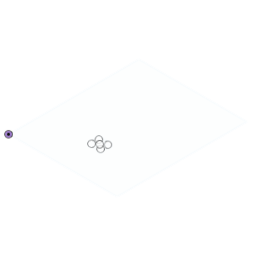
designing_cuts_acrylic_plates (Autodesk Fusion 360 design; units mm, degrees)
part number: 2026-05-25-10-10-53-826
Autodesk Fusion 360 part; units mm, degrees
sketch "Sketch3" plane through (0, 0, 0) normal (0, 0, 1) x (1, 0, 0)
  line L0 (0, 0) -> (225, 0)
  line L1 (225, 0) -> (225, 405)
  line L2 (225, 405) -> (0, 405)
  line L3 (0, 405) -> (0, 0)
  dimension "d6" = 225
  dimension "d7" = 405
  constraint horizontal L0
  constraint vertical L1
  constraint horizontal L2
  constraint vertical L3
  constraint coincident L0.start L3.end
  measures "d6" distance of L1 L3
  measures "d7" distance of L0 L2
sketch "Sketch4" plane through (0, 0, 0) normal (0, 0, 1) x (1, 0, 0)
  line L0 (0, 0) -> (75, 0)
  line L1 (75, 0) -> (75, 81)
  line L2 (75, 81) -> (0, 81)
  line L3 (0, 81) -> (0, 0)
  dimension "d8" = 75
  dimension "d9" = 81
  constraint horizontal L0
  constraint vertical L1
  constraint horizontal L2
  constraint vertical L3
  constraint coincident L0.start L3.end
  measures "d8" distance of L1 L3
  measures "d9" distance of L0 L2
extrude "Extrude1" add sketch "Sketch3" along normal blind 3 makes body 1
sketch "Sketch5" plane through (0, 0, 0) normal (0, 0, 1) x (1, 0, 0)
  line L0 (0, 0) -> (225, 0) construction
  line L1 (225, 0) -> (225, 405) construction
  line L2 (225, 405) -> (0, 405) construction
  line L3 (0, 405) -> (0, 0) construction
  line L4 (0, 81) -> (225, 81) construction
  line L5 (0, 162) -> (225, 162) construction
  line L6 (0, 243) -> (225, 243) construction
  line L7 (0, 324) -> (225, 324) construction
  line L8 (150, 405) -> (150, 0) construction
  line L9 (75, 405) -> (75, 0) construction
  line L10 (22.5, 388.5) -> (52.5, 388.5) construction
  line L11 (52.5, 388.5) -> (52.5, 340.5) construction
  line L12 (52.5, 340.5) -> (22.5, 340.5) construction
  line L13 (22.5, 340.5) -> (22.5, 388.5) construction
  line L14 (127.5, 388.5) -> (127.5, 340.5) construction
  line L15 (97.5, 388.5) -> (127.5, 388.5) construction
  line L16 (97.5, 340.5) -> (97.5, 388.5) construction
  line L17 (127.5, 340.5) -> (97.5, 340.5) construction
  line L18 (202.5, 388.5) -> (202.5, 340.5) construction
  line L19 (172.5, 388.5) -> (202.5, 388.5) construction
  line L20 (172.5, 340.5) -> (172.5, 388.5) construction
  line L21 (202.5, 340.5) -> (172.5, 340.5) construction
  line L22 (22.5, 226.5) -> (52.5, 226.5) construction
  line L23 (22.5, 178.5) -> (22.5, 226.5) construction
  line L24 (52.5, 226.5) -> (52.5, 178.5) construction
  line L25 (52.5, 178.5) -> (22.5, 178.5) construction
  line L26 (97.5, 226.5) -> (127.5, 226.5) construction
  line L27 (97.5, 178.5) -> (97.5, 226.5) construction
  line L28 (127.5, 226.5) -> (127.5, 178.5) construction
  line L29 (127.5, 178.5) -> (97.5, 178.5) construction
  line L30 (172.5, 226.5) -> (202.5, 226.5) construction
  line L31 (172.5, 178.5) -> (172.5, 226.5) construction
  line L32 (202.5, 226.5) -> (202.5, 178.5) construction
  line L33 (202.5, 178.5) -> (172.5, 178.5) construction
  line L34 (22.5, 64.5) -> (52.5, 64.5) construction
  line L35 (22.5, 16.5) -> (22.5, 64.5) construction
  line L36 (52.5, 64.5) -> (52.5, 16.5) construction
  line L37 (52.5, 16.5) -> (22.5, 16.5) construction
  line L38 (97.5, 64.5) -> (127.5, 64.5) construction
  line L39 (97.5, 16.5) -> (97.5, 64.5) construction
  line L40 (127.5, 64.5) -> (127.5, 16.5) construction
  line L41 (127.5, 16.5) -> (97.5, 16.5) construction
  line L42 (172.5, 64.5) -> (202.5, 64.5) construction
  line L43 (172.5, 16.5) -> (172.5, 64.5) construction
  line L44 (202.5, 64.5) -> (202.5, 16.5) construction
  line L45 (202.5, 16.5) -> (172.5, 16.5) construction
  line L46 (52.5, 307.5) -> (52.5, 259.5) construction
  line L47 (22.5, 307.5) -> (52.5, 307.5) construction
  line L48 (22.5, 259.5) -> (22.5, 307.5) construction
  line L49 (52.5, 259.5) -> (22.5, 259.5) construction
  line L50 (97.5, 307.5) -> (127.5, 307.5) construction
  line L51 (127.5, 307.5) -> (127.5, 259.5) construction
  line L52 (97.5, 259.5) -> (97.5, 307.5) construction
  line L53 (127.5, 259.5) -> (97.5, 259.5) construction
  line L54 (172.5, 307.5) -> (202.5, 307.5) construction
  line L55 (172.5, 259.5) -> (172.5, 307.5) construction
  line L56 (202.5, 307.5) -> (202.5, 259.5) construction
  line L57 (202.5, 259.5) -> (172.5, 259.5) construction
  line L58 (22.5, 145.5) -> (52.5, 145.5) construction
  line L59 (22.5, 97.5) -> (22.5, 145.5) construction
  line L60 (52.5, 145.5) -> (52.5, 97.5) construction
  line L61 (52.5, 97.5) -> (22.5, 97.5) construction
  line L62 (97.5, 145.5) -> (127.5, 145.5) construction
  line L63 (97.5, 97.5) -> (97.5, 145.5) construction
  line L64 (127.5, 145.5) -> (127.5, 97.5) construction
  line L65 (127.5, 97.5) -> (97.5, 97.5) construction
  line L66 (172.5, 97.5) -> (172.5, 145.5) construction
  line L67 (172.5, 145.5) -> (202.5, 145.5) construction
  line L68 (202.5, 145.5) -> (202.5, 97.5) construction
  line L69 (202.5, 97.5) -> (172.5, 97.5) construction
  line L70 (22.5, 348.5) -> (52.5, 348.5) construction
  line L71 (25, 340.5) -> (50, 340.5) construction
  line L72 (50, 340.5) -> (50, 372) construction
  line L73 (50, 372) -> (25, 372) construction
  line L74 (25, 372) -> (25, 340.5) construction
  line L75 (26, 358.5) -> (47, 358.5) construction
  line L76 (47, 358.5) -> (47, 341.5) construction
  line L77 (47, 341.5) -> (26, 341.5) construction
  line L78 (26, 341.5) -> (26, 358.5) construction
  line L79 (125, 372) -> (100, 372) construction
  line L80 (100, 372) -> (100, 340.5) construction
  line L81 (125, 340.5) -> (125, 372) construction
  line L82 (122, 358.5) -> (122, 341.5) construction
  line L83 (101, 358.5) -> (122, 358.5) construction
  line L84 (101, 341.5) -> (101, 358.5) construction
  line L85 (122, 341.5) -> (101, 341.5) construction
  line L86 (97.5, 348.5) -> (127.5, 348.5) construction
  line L87 (200, 372) -> (175, 372) construction
  line L88 (175, 372) -> (175, 340.5) construction
  line L89 (200, 340.5) -> (200, 372) construction
  line L90 (197, 358.5) -> (197, 341.5) construction
  line L91 (176, 358.5) -> (197, 358.5) construction
  line L92 (176, 341.5) -> (176, 358.5) construction
  line L93 (197, 341.5) -> (176, 341.5) construction
  line L94 (172.5, 348.5) -> (202.5, 348.5) construction
  line L95 (200, 291) -> (175, 291) construction
  line L96 (176, 277.5) -> (197, 277.5) construction
  line L97 (175, 291) -> (175, 259.5) construction
  line L98 (200, 259.5) -> (200, 291) construction
  line L99 (197, 277.5) -> (197, 260.5) construction
  line L100 (176, 260.5) -> (176, 277.5) construction
  line L101 (197, 260.5) -> (176, 260.5) construction
  line L102 (172.5, 267.5) -> (202.5, 267.5) construction
  line L103 (101, 277.5) -> (122, 277.5) construction
  line L104 (122, 277.5) -> (122, 260.5) construction
  line L105 (122, 260.5) -> (101, 260.5) construction
  line L106 (101, 260.5) -> (101, 277.5) construction
  line L107 (125, 291) -> (100, 291) construction
  line L108 (125, 259.5) -> (125, 291) construction
  line L109 (100, 291) -> (100, 259.5) construction
  line L110 (97.5, 267.5) -> (127.5, 267.5) construction
  line L111 (50, 291) -> (25, 291) construction
  line L112 (25, 291) -> (25, 259.5) construction
  line L113 (50, 259.5) -> (50, 291) construction
  line L114 (26, 277.5) -> (47, 277.5) construction
  line L115 (26, 260.5) -> (26, 277.5) construction
  line L116 (47, 277.5) -> (47, 260.5) construction
  line L117 (22.5, 267.5) -> (52.5, 267.5) construction
  line L118 (47, 260.5) -> (26, 260.5) construction
  line L119 (200, 210) -> (175, 210) construction
  line L120 (176, 196.5) -> (197, 196.5) construction
  line L121 (175, 210) -> (175, 178.5) construction
  line L122 (200, 178.5) -> (200, 210) construction
  line L123 (197, 196.5) -> (197, 179.5) construction
  line L124 (176, 179.5) -> (176, 196.5) construction
  line L125 (197, 179.5) -> (176, 179.5) construction
  line L126 (172.5, 186.5) -> (202.5, 186.5) construction
  line L127 (101, 196.5) -> (122, 196.5) construction
  line L128 (122, 196.5) -> (122, 179.5) construction
  line L129 (122, 179.5) -> (101, 179.5) construction
  line L130 (101, 179.5) -> (101, 196.5) construction
  line L131 (125, 210) -> (100, 210) construction
  line L132 (125, 178.5) -> (125, 210) construction
  line L133 (100, 210) -> (100, 178.5) construction
  line L134 (97.5, 186.5) -> (127.5, 186.5) construction
  line L135 (50, 210) -> (25, 210) construction
  line L136 (25, 210) -> (25, 178.5) construction
  line L137 (50, 178.5) -> (50, 210) construction
  line L138 (26, 196.5) -> (47, 196.5) construction
  line L139 (26, 179.5) -> (26, 196.5) construction
  line L140 (47, 196.5) -> (47, 179.5) construction
  line L141 (22.5, 186.5) -> (52.5, 186.5) construction
  line L142 (47, 179.5) -> (26, 179.5) construction
  line L143 (200, 129) -> (175, 129) construction
  line L144 (176, 115.5) -> (197, 115.5) construction
  line L145 (175, 129) -> (175, 97.5) construction
  line L146 (200, 97.5) -> (200, 129) construction
  line L147 (197, 115.5) -> (197, 98.5) construction
  line L148 (176, 98.5) -> (176, 115.5) construction
  line L149 (197, 98.5) -> (176, 98.5) construction
  line L150 (172.5, 105.5) -> (202.5, 105.5) construction
  line L151 (101, 115.5) -> (122, 115.5) construction
  line L152 (122, 115.5) -> (122, 98.5) construction
  line L153 (122, 98.5) -> (101, 98.5) construction
  line L154 (101, 98.5) -> (101, 115.5) construction
  line L155 (125, 129) -> (100, 129) construction
  line L156 (125, 97.5) -> (125, 129) construction
  line L157 (100, 129) -> (100, 97.5) construction
  line L158 (97.5, 105.5) -> (127.5, 105.5) construction
  line L159 (50, 129) -> (25, 129) construction
  line L160 (25, 129) -> (25, 97.5) construction
  line L161 (50, 97.5) -> (50, 129) construction
  line L162 (26, 115.5) -> (47, 115.5) construction
  line L163 (26, 98.5) -> (26, 115.5) construction
  line L164 (47, 115.5) -> (47, 98.5) construction
  line L165 (22.5, 105.5) -> (52.5, 105.5) construction
  line L166 (47, 98.5) -> (26, 98.5) construction
  line L167 (200, 48) -> (175, 48) construction
  line L168 (176, 34.5) -> (197, 34.5) construction
  line L169 (175, 48) -> (175, 16.5) construction
  line L170 (200, 16.5) -> (200, 48) construction
  line L171 (197, 34.5) -> (197, 17.5) construction
  line L172 (176, 17.5) -> (176, 34.5) construction
  line L173 (197, 17.5) -> (176, 17.5) construction
  line L174 (172.5, 24.5) -> (202.5, 24.5) construction
  line L175 (101, 34.5) -> (122, 34.5) construction
  line L176 (122, 34.5) -> (122, 17.5) construction
  line L177 (122, 17.5) -> (101, 17.5) construction
  line L178 (101, 17.5) -> (101, 34.5) construction
  line L179 (125, 48) -> (100, 48) construction
  line L180 (125, 16.5) -> (125, 48) construction
  line L181 (100, 48) -> (100, 16.5) construction
  line L182 (97.5, 24.5) -> (127.5, 24.5) construction
  line L183 (50, 48) -> (25, 48) construction
  line L184 (25, 48) -> (25, 16.5) construction
  line L185 (50, 16.5) -> (50, 48) construction
  line L186 (26, 34.5) -> (47, 34.5) construction
  line L187 (26, 17.5) -> (26, 34.5) construction
  line L188 (47, 34.5) -> (47, 17.5) construction
  line L189 (22.5, 24.5) -> (52.5, 24.5) construction
  line L190 (47, 17.5) -> (26, 17.5) construction
  dimension "d12" = 225
  dimension "d13" = 405
  dimension "d14" = 81
  dimension "d17" = 0
  dimension "d18" = 162
  dimension "d21" = 0
  dimension "d22" = 81
  dimension "d23" = 75
  dimension "d24" = 75
  dimension "d25" = 30
  dimension "d26" = 48
  dimension "d27" = 16.5
  dimension "d28" = 22.5
  dimension "d31" = 150
  dimension "d32" = 0
  dimension "d35" = 0
  dimension "d36" = -324
  dimension "d39" = 0
  dimension "d40" = 81
  dimension "d43" = 0
  dimension "d44" = -81
  dimension "d45" = 8
  dimension "d46" = 25
  dimension "d47" = 31.5
  dimension "d48" = 2.5
  dimension "d49" = 21
  dimension "d50" = 17
  dimension "d51" = 1
  dimension "d52" = 1
  dimension "d55" = 150
  dimension "d56" = 0
  dimension "d59" = 0
  dimension "d60" = -324
  constraint coincident L0.start L3.end
  constraint horizontal L0
  constraint perpendicular L0 L1
  constraint perpendicular L1 L2
  constraint perpendicular L0 L3
  constraint coincident L3 L4.start
  constraint coincident L1 L4.end
  constraint perpendicular L1 L4
  constraint coincident L2 L8.start
  constraint coincident L0 L8.end
  constraint perpendicular L0 L8
  constraint coincident L2 L9.start
  constraint coincident L0 L9.end
  constraint perpendicular L0 L9
  constraint horizontal L10
  constraint vertical L11
  constraint horizontal L12
  constraint vertical L13
  constraint coincident L13 L70.start
  constraint coincident L11 L70.end
  constraint perpendicular L11 L70
  constraint horizontal L71
  constraint vertical L72
  constraint horizontal L73
  constraint vertical L74
  constraint coincident L12 L71.start
  constraint horizontal L75
  constraint vertical L76
  constraint horizontal L77
  constraint vertical L78
  measures "d12" distance of L0.start L0.end
  measures "d13" distance of L0.end L1.end
  measures "d14" distance of L0 L4
  measures "d23" distance of L1 L8
  measures "d24" distance of L3 L9
  measures "d25" distance of L10.start L10.end
  measures "d26" distance of L10 L12
  measures "d27" distance of L2 L10
  measures "d28" distance of L3 L13
  measures "d45" distance of L12 L70
  measures "d46" distance of L72 L74
  measures "d47" distance of L71 L73
  measures "d48" distance of L11 L72
  measures "d49" distance of L76 L78
  measures "d50" distance of L75 L77
  measures "d51" distance of L74 L78
  measures "d52" distance of L12 L77
sketch "Sketch6" plane through (0, 0, 0) normal (0, 0, 1) x (1, 0, 0)
  line L0 (0, 0) -> (225, 0)
  line L1 (225, 0) -> (225, 405)
  line L2 (225, 405) -> (0, 405)
  line L3 (0, 405) -> (0, 0)
  line L4 (197, 358.5) -> (176, 358.5)
  line L5 (176, 358.5) -> (176, 341.5)
  line L6 (176, 341.5) -> (197, 341.5)
  line L7 (197, 341.5) -> (197, 358.5)
  line L8 (98.5, 361) -> (124.5, 361)
  line L9 (124.5, 361) -> (124.5, 339)
  line L10 (124.5, 339) -> (98.5, 339)
  line L11 (98.5, 339) -> (98.5, 361)
  line L12 (122, 358.5) -> (122, 341.5)
  line L13 (101, 358.5) -> (122, 358.5)
  line L14 (26, 363.5) -> (47, 363.5)
  line L15 (52, 358.5) -> (52, 341.5)
  line L16 (47, 336.5) -> (26, 336.5)
  line L17 (21, 341.5) -> (21, 358.5)
  line L18 (26, 358.5) -> (47, 358.5)
  line L19 (47, 358.5) -> (47, 341.5)
  arc A0 (26, 363.5) -> (21, 358.5) centre (26, 358.5) ccw
  arc A1 (52, 358.5) -> (47, 363.5) centre (47, 358.5) ccw
  arc A2 (21, 341.5) -> (26, 336.5) centre (26, 341.5) ccw
  arc A3 (47, 336.5) -> (52, 341.5) centre (47, 341.5) ccw
  line L20 (171.5, 308.5) -> (203.5, 308.5)
  line L21 (203.5, 308.5) -> (203.5, 258.5)
  line L22 (203.5, 258.5) -> (171.5, 258.5)
  line L23 (171.5, 258.5) -> (171.5, 308.5)
  line L24 (172.5, 307.5) -> (202.5, 307.5)
  line L25 (202.5, 307.5) -> (202.5, 259.5)
  circle A4 centre (111.5, 269) radius 7.5
  line L26 (122, 277.5) -> (122, 260.5)
  line L27 (101, 277.5) -> (122, 277.5)
  line L28 (21, 277.5) -> (52, 277.5)
  line L29 (52, 277.5) -> (52, 260.5)
  line L30 (52, 260.5) -> (21, 260.5)
  line L31 (21, 260.5) -> (21, 277.5)
  line L32 (47, 260.5) -> (26, 260.5)
  line L33 (26, 260.5) -> (26, 277.5)
  line L34 (22.4805, 198.9951) -> (26.4805, 198.9951)
  line L35 (28.4805, 198.9951) -> (32.4805, 198.9951)
  line L36 (34.4805, 198.9951) -> (38.4805, 198.9951)
  line L37 (40.4805, 198.9951) -> (44.4805, 198.9951)
  line L38 (46.4805, 198.9951) -> (50.4805, 198.9951)
  line L39 (50.4805, 198.9951) -> (50.4805, 194.9951)
  line L40 (46.4805, 194.9951) -> (46.4805, 198.9951)
  line L41 (44.4805, 198.9951) -> (44.4805, 194.9951)
  line L42 (40.4805, 194.9951) -> (40.4805, 198.9951)
  line L43 (38.4805, 198.9951) -> (38.4805, 194.9951)
  line L44 (34.4805, 194.9951) -> (34.4805, 198.9951)
  line L45 (32.4805, 198.9951) -> (32.4805, 194.9951)
  line L46 (28.4805, 194.9951) -> (28.4805, 198.9951)
  line L47 (26.4805, 198.9951) -> (26.4805, 194.9951)
  line L48 (22.4805, 194.9951) -> (22.4805, 198.9951)
  line L49 (26.4805, 194.9951) -> (22.4805, 194.9951)
  line L50 (32.4805, 194.9951) -> (28.4805, 194.9951)
  line L51 (38.4805, 194.9951) -> (34.4805, 194.9951)
  line L52 (44.4805, 194.9951) -> (40.4805, 194.9951)
  line L53 (50.4805, 194.9951) -> (46.4805, 194.9951)
  line L54 (22.4805, 192.9951) -> (26.4805, 192.9951)
  line L55 (28.4805, 192.9951) -> (32.4805, 192.9951)
  line L56 (34.4805, 192.9951) -> (38.4805, 192.9951)
  line L57 (40.4805, 192.9951) -> (44.4805, 192.9951)
  line L58 (46.4805, 192.9951) -> (50.4805, 192.9951)
  line L59 (50.4805, 192.9951) -> (50.4805, 188.9951)
  line L60 (46.4805, 188.9951) -> (46.4805, 192.9951)
  line L61 (44.4805, 192.9951) -> (44.4805, 188.9951)
  line L62 (40.4805, 188.9951) -> (40.4805, 192.9951)
  line L63 (38.4805, 192.9951) -> (38.4805, 188.9951)
  line L64 (34.4805, 188.9951) -> (34.4805, 192.9951)
  line L65 (32.4805, 192.9951) -> (32.4805, 188.9951)
  line L66 (28.4805, 188.9951) -> (28.4805, 192.9951)
  line L67 (26.4805, 192.9951) -> (26.4805, 188.9951)
  line L68 (22.4805, 188.9951) -> (22.4805, 192.9951)
  line L69 (26.4805, 188.9951) -> (22.4805, 188.9951)
  line L70 (32.4805, 188.9951) -> (28.4805, 188.9951)
  line L71 (38.4805, 188.9951) -> (34.4805, 188.9951)
  line L72 (44.4805, 188.9951) -> (40.4805, 188.9951)
  line L73 (50.4805, 188.9951) -> (46.4805, 188.9951)
  line L74 (22.4805, 186.9951) -> (26.4805, 186.9951)
  line L75 (28.4805, 186.9951) -> (32.4805, 186.9951)
  line L76 (34.4805, 186.9951) -> (38.4805, 186.9951)
  line L77 (40.4805, 186.9951) -> (44.4805, 186.9951)
  line L78 (46.4805, 186.9951) -> (50.4805, 186.9951)
  line L79 (50.4805, 186.9951) -> (50.4805, 182.9951)
  line L80 (46.4805, 182.9951) -> (46.4805, 186.9951)
  line L81 (44.4805, 186.9951) -> (44.4805, 182.9951)
  line L82 (40.4805, 182.9951) -> (40.4805, 186.9951)
  line L83 (38.4805, 186.9951) -> (38.4805, 182.9951)
  line L84 (34.4805, 182.9951) -> (34.4805, 186.9951)
  line L85 (32.4805, 186.9951) -> (32.4805, 182.9951)
  line L86 (28.4805, 182.9951) -> (28.4805, 186.9951)
  line L87 (26.4805, 186.9951) -> (26.4805, 182.9951)
  line L88 (22.4805, 182.9951) -> (22.4805, 186.9951)
  line L89 (26.4805, 182.9951) -> (22.4805, 182.9951)
  line L90 (32.4805, 182.9951) -> (28.4805, 182.9951)
  line L91 (38.4805, 182.9951) -> (34.4805, 182.9951)
  line L92 (44.4805, 182.9951) -> (40.4805, 182.9951)
  line L93 (50.4805, 182.9951) -> (46.4805, 182.9951)
  line L94 (22.4805, 180.9951) -> (26.4805, 180.9951)
  line L95 (28.4805, 180.9951) -> (32.4805, 180.9951)
  line L96 (34.4805, 180.9951) -> (38.4805, 180.9951)
  line L97 (40.4805, 180.9951) -> (44.4805, 180.9951)
  line L98 (46.4805, 180.9951) -> (50.4805, 180.9951)
  line L99 (50.4805, 180.9951) -> (50.4805, 176.9951)
  line L100 (46.4805, 176.9951) -> (46.4805, 180.9951)
  line L101 (44.4805, 180.9951) -> (44.4805, 176.9951)
  line L102 (40.4805, 176.9951) -> (40.4805, 180.9951)
  line L103 (38.4805, 180.9951) -> (38.4805, 176.9951)
  line L104 (34.4805, 176.9951) -> (34.4805, 180.9951)
  line L105 (32.4805, 180.9951) -> (32.4805, 176.9951)
  line L106 (28.4805, 176.9951) -> (28.4805, 180.9951)
  line L107 (26.4805, 180.9951) -> (26.4805, 176.9951)
  line L108 (22.4805, 176.9951) -> (22.4805, 180.9951)
  line L109 (26.4805, 176.9951) -> (22.4805, 176.9951)
  line L110 (32.4805, 176.9951) -> (28.4805, 176.9951)
  line L111 (38.4805, 176.9951) -> (34.4805, 176.9951)
  line L112 (44.4805, 176.9951) -> (40.4805, 176.9951)
  line L113 (50.4805, 176.9951) -> (46.4805, 176.9951)
  line L114 (25, 210) -> (25, 178.5) construction
  line L115 (97.5, 178.5) -> (97.5, 226.5) construction
  arc A5 (193.5603, 181.2758) -> (193.5603, 194.7241) centre (186.5, 188) ccw
  arc A6 (189.9397, 184.7241) -> (189.9396, 191.2759) centre (186.5, 188) ccw
  arc A7 (193.5603, 194.7241) -> (189.9396, 191.2759) centre (191.75, 193) ccw
  arc A8 (189.9397, 184.7241) -> (193.5603, 181.2758) centre (191.75, 183) ccw
  arc A9 (179.4397, 194.7241) -> (179.4397, 181.2758) centre (186.5, 188) ccw
  arc A10 (179.4397, 181.2758) -> (183.0603, 184.7241) centre (181.25, 183) ccw
  arc A11 (183.0603, 191.2758) -> (183.0603, 184.7241) centre (186.5, 188) ccw
  arc A12 (183.0603, 191.2758) -> (179.4397, 194.7241) centre (181.25, 193) ccw
  line L116 (22.4805, 198.9951) -> (50.4805, 176.9951) construction
  line L117 (50.4805, 198.9951) -> (22.4805, 176.9951) construction
  line L118 (26, 196.5) -> (47, 179.5) construction
  line L119 (47, 196.5) -> (26, 179.5) construction
  line L120 (122, 196.5) -> (122, 179.5)
  line L121 (99, 195.5) -> (124, 195.5)
  line L122 (124, 195.5) -> (124, 189.5)
  line L123 (124, 189.5) -> (99, 189.5)
  line L124 (99, 189.5) -> (99, 195.5)
  line L125 (124, 180.5) -> (99, 180.5)
  line L126 (124, 186.5) -> (124, 180.5)
  line L127 (99, 186.5) -> (124, 186.5)
  line L128 (99, 180.5) -> (99, 186.5)
  line L129 (122, 179.5) -> (101, 179.5)
  dimension "d61" = 225
  dimension "d62" = 405
  dimension "d63" = 17
  dimension "d64" = 21
  dimension "d65" = 28
  dimension "d66" = 46.5
  dimension "d67" = 26
  dimension "d68" = 22
  dimension "d69" = 2.5
  dimension "d70" = 2.5
  dimension "d71" = 31
  dimension "d72" = 27
  dimension "d73" = 5
  dimension "d74" = 5
  dimension "d75" = 5
  dimension "d76" = 32
  dimension "d77" = 50
  dimension "d78" = 1
  dimension "d79" = 1
  dimension "d80" = 15
  dimension "d81" = 10.5
  dimension "d82" = 8.5
  dimension "d83" = 31
  dimension "d84" = 17
  dimension "d85" = 17
  dimension "d86" = 5
  dimension "d116" = 10
  dimension "d120" = 360
  dimension "d123" = 2.5
  dimension "d124" = 2.5
  dimension "d129" = 25
  dimension "d130" = 6
  dimension "d131" = 2
  dimension "d134" = 0
  dimension "d135" = -9
  dimension "d136" = 1
  constraint horizontal L0
  constraint vertical L1
  constraint horizontal L2
  constraint vertical L3
  constraint coincident L0.start L3.end
  constraint horizontal L4
  constraint vertical L5
  constraint horizontal L6
  constraint vertical L7
  constraint horizontal L8
  constraint vertical L9
  constraint horizontal L10
  constraint vertical L11
  constraint horizontal L14
  constraint vertical L15
  constraint horizontal L16
  constraint vertical L17
  constraint tangent L14 A0
  constraint tangent L17 A0
  constraint tangent L14 A1
  constraint tangent L15 A1
  constraint equal A0 A1
  constraint tangent L16 A2
  constraint tangent L17 A2
  constraint equal A0 A2
  constraint tangent L15 A3
  constraint tangent L16 A3
  constraint equal A0 A3
  constraint horizontal L20
  constraint vertical L21
  constraint horizontal L22
  constraint vertical L23
  constraint horizontal L28
  constraint vertical L29
  constraint horizontal L30
  constraint vertical L31
  constraint horizontal L121
  constraint vertical L122
  constraint horizontal L123
  constraint vertical L124
  measures "d61" distance of L1 L3
  measures "d62" distance of L0 L2
  measures "d63" distance of L4 L6
  measures "d64" distance of L5 L7
  measures "d65" distance of L1 L7
  measures "d66" distance of L2 L4
  measures "d67" distance of L9 L11
  measures "d68" distance of L8 L10
  measures "d69" distance of L9 L12
  measures "d70" distance of L8 L13
  measures "d71" distance of L15 L17
  measures "d72" distance of L14 L16
  measures "d73" distance of L14 L18
  measures "d74" distance of L15 L19
  measures "d75" radius of A0
  measures "d76" distance of L21 L23
  measures "d77" distance of L20 L22
  measures "d78" distance of L20 L24
  measures "d79" distance of L21 L25
  measures "d80" diameter of A4
  measures "d81" distance of A4.centre L26
  measures "d82" distance of A4.centre L27
  measures "d83" distance of L28.start L28.end
  measures "d84" distance of L28 L30
  measures "d85" distance of L28 L32
  measures "d86" distance of L31 L33
  measures "d116" distance of A7.centre A8.centre
  measures "d123" radius of A12
  measures "d124" radius of A10
  measures "d129" distance of L121.start L121.end
  measures "d130" distance of L121.start L123.end
  measures "d131" distance of L120 L122
  measures "d136" distance of L125 L129
sketch "Sketch7" plane through (0, 0, 0) normal (0, 0, 1) x (1, 0, 0)
  spline S0 degree 5 poles (160, 199) (160.9519, 200.1243) (162.8063, 202.1939) (165.4397, 204.7612) (168.6855, 207.174) (172.4676, 208.8335) (176.1709, 209.508) (179.9682, 209.5107) (183.953, 209) (188.0845, 207.8917) (192.2444, 205.9499) (195.4768, 203.4877) (197.7892, 201.0065) (199.2727, 199.0522) (200, 198) knots 0 0 0 0 0 0 0.1 0.2 0.3 0.4 0.5 0.6 0.7 0.8 0.9 1 1 1 1 1 1
  line L0 (196.7637, 202.6821) -> (203.2363, 193.3179)
  line L1 (155.6402, 193.8507) -> (164.3598, 204.1493)
  spline S1 degree 5 poles (163.8148, 196.5618) (164.3055, 197.3339) (165.3314, 198.7748) (167.0036, 200.6266) (169.4748, 202.505) (172.8325, 204.0096) (176.2999, 204.8254) (179.7341, 205.0754) (183.0505, 204.8116) (186.2635, 203.9837) (189.4452, 202.4735) (192.0421, 200.5997) (194.0574, 198.7584) (195.4365, 197.3278) (196.1349, 196.5618) knots 0 0 0 0 0 0 0.1 0.2 0.3 0.4 0.5 0.6 0.7 0.8 0.9 1 1 1 1 1 1
  line L2 (193, 200) -> (199.2698, 193.1236)
  line L3 (161.6297, 193.1236) -> (166, 200)
  arc A0 (160, 199) -> (163.8148, 196.5618) centre (161.9043, 197.7761) ccw
  arc A1 (196.1349, 196.5618) -> (200, 198) centre (197.9174, 197.6842) ccw
  line L4 (179.8701, 209.3892) -> (179.8701, 204.9451)
  arc A2 (109.1067, 244.7264) -> (64.1067, 244.7264) centre (86.6067, 230.5097) ccw
  arc A3 (112.4883, 246.8631) -> (60.7252, 246.8631) centre (86.6067, 230.5097) ccw
  arc A4 (60.7252, 246.8631) -> (64.1067, 244.7264) centre (62.416, 245.7948) ccw
  arc A5 (109.1067, 244.7264) -> (112.4883, 246.8631) centre (110.7975, 245.7948) ccw
  arc A6 (48, 308) -> (11.108, 308.0557) centre (29.5227, 287.2694) ccw
  arc A7 (48, 300) -> (11.108, 300.0557) centre (29.5227, 279.2694) ccw
  arc A8 (48, 292) -> (11.108, 292.0557) centre (29.5227, 271.2694) ccw
  point P0 (179.8701, 209.3892)
  point P1 (179.5347, 204.9458)
  dimension "d109" = 4
  dimension "d112" = 0
  dimension "d113" = -16
  constraint midpoint S0.end L0
  constraint midpoint S0.start L1
  constraint midpoint S1.end L2
  constraint midpoint S1.start L3
  constraint tangent L3 A0
  constraint coincident P0 L4.start
  constraint coincident S1 L4.end
  constraint vertical L4
extrude "Extrude2" add sketch "Sketch6" along normal blind 3 separate body contours L0 L1 L2 L3 | A5 A6 A7 A8 | A9 A10 A11 A12 | L120 L121 L122 L123 | L120 L121 L123 L124 | L120 L125 L126 L127 | L120 L125 L127 L128 makes body 2
extrude "Extrude3" add sketch "Sketch6" along normal blind 3 separate body contours L0 L1 L2 L3 | L120 L121 L122 L123 | L120 L121 L123 L124 | L120 L125 L126 L127 | L120 L125 L127 L128 makes body 3
extrude "Extrude4" add sketch "Sketch6" along normal blind 3 separate body makes body 4
sketch "Sketch8" plane through (0, 0, 0) normal (0, 0, 1) x (1, 0, 0)
  line L0 (0, 0) -> (250, 0)
  line L1 (250, 0) -> (250, 300)
  line L2 (250, 300) -> (0, 300)
  line L3 (0, 300) -> (0, 0)
  arc A0 (132.0603, 56.7241) -> (128.4396, 53.2759) centre (130.25, 55) ccw
  arc A1 (132.0603, 43.2758) -> (132.0603, 56.7241) centre (125, 50) ccw
  arc A2 (128.4397, 46.7241) -> (128.4396, 53.2759) centre (125, 50) ccw
  arc A3 (128.4397, 46.7241) -> (132.0603, 43.2758) centre (130.25, 45) ccw
  arc A4 (117.9397, 43.2759) -> (121.5604, 46.7241) centre (119.75, 45) ccw
  arc A5 (121.5603, 53.2759) -> (121.5604, 46.7241) centre (125, 50) ccw
  arc A6 (121.5603, 53.2759) -> (117.9397, 56.7242) centre (119.75, 55) ccw
  arc A7 (117.9397, 56.7242) -> (117.9397, 43.2759) centre (125, 50) ccw
  point P0 (125, 50)
  dimension "d139" = 250
  dimension "d140" = 300
  dimension "d144" = 360
  dimension "d145" = 10
  dimension "d146" = 2.5
  dimension "d147" = 2.5
  dimension "d148" = 50
  dimension "d149" = 125
  constraint horizontal L0
  constraint vertical L1
  constraint horizontal L2
  constraint vertical L3
  constraint coincident L0.start L3.end
  measures "d139" distance of L0.start L0.end
  measures "d140" distance of L0 L2
  measures "d145" distance of A0.centre A3.centre
  measures "d146" radius of A6
  measures "d147" radius of A4
  measures "d148" distance of L0 P0
  measures "d149" distance of L3 P0
sketch "Sketch9" plane through (0, 0, 0) normal (0, 0, 1) x (1, 0, 0)
  line L0 (0, 0) -> (250, 0)
  line L1 (250, 0) -> (250, 300)
  line L2 (250, 300) -> (0, 300)
  line L3 (0, 300) -> (0, 0)
  line L4 (114.5, 98.5) -> (135.5, 98.5)
  line L5 (140.5, 93.5) -> (140.5, 76.5)
  line L6 (135.5, 71.5) -> (114.5, 71.5)
  line L7 (109.5, 76.5) -> (109.5, 93.5)
  arc A0 (114.5, 98.5) -> (109.5, 93.5) centre (114.5, 93.5) ccw
  arc A1 (109.5, 76.5) -> (114.5, 71.5) centre (114.5, 76.5) ccw
  arc A2 (135.5, 71.5) -> (140.5, 76.5) centre (135.5, 76.5) ccw
  arc A3 (140.5, 93.5) -> (135.5, 98.5) centre (135.5, 93.5) ccw
  point P0 (125, 85)
  dimension "d141" = 300
  dimension "d142" = 250
  dimension "d156" = 31
  dimension "d157" = 27
  dimension "d158" = 5
  dimension "d159" = 5
  dimension "d160" = 15.5
  dimension "d161" = 13.5
  dimension "d162" = 85
  dimension "d163" = 125
  constraint horizontal L0
  constraint vertical L1
  constraint horizontal L2
  constraint vertical L3
  constraint coincident L0.start L3.end
  constraint horizontal L4
  constraint vertical L5
  constraint horizontal L6
  constraint vertical L7
  constraint tangent L7 A0
  constraint tangent L4 A0
  constraint tangent L7 A1
  constraint tangent L6 A1
  constraint tangent L5 A2
  constraint tangent L6 A2
  constraint equal A1 A2
  constraint tangent L5 A3
  constraint tangent L4 A3
  constraint equal A1 A3
  measures "d141" distance of L0.start L2.end
  measures "d142" distance of L1 L3
  measures "d156" distance of L5 L7
  measures "d157" distance of L4 L6
  measures "d158" radius of A0
  measures "d159" radius of A1
  measures "d160" distance of L5 P0
  measures "d161" distance of L4 P0
  measures "d162" distance of L0 P0
  measures "d163" distance of L1 P0
hidden bodies 1 2 3 4
